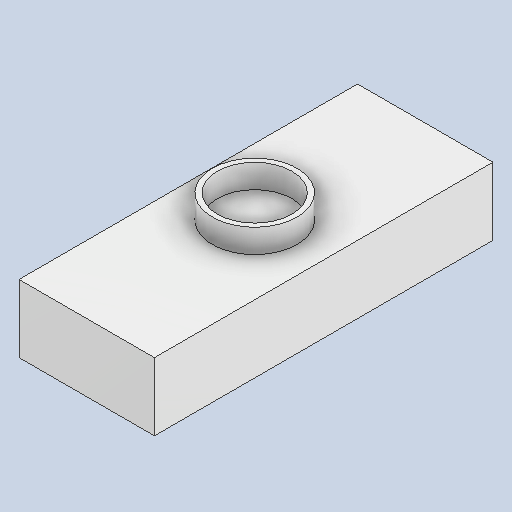
# Autodesk Inventor part: Suporte para estrutura_CPY_CPY1
Saved by Autodesk Inventor 2024 (Build 280153000, 153)
## iProperties
Created: 2024-05-09
Part Number: Suporte para estrutura_CPY_CPY1
Material: ABS plástico
Document SubType Name: Modeling
Designer: mathe
Density: 1.06 g/cm^3
Appearance: Suave - Branco
Author: mathe
Autodesk Inventor part; units mm, degrees
ref_plane "YZ Plane" through (0, 0, 0) normal (1, 0, 0) x (0, 1, 0)
ref_plane "XZ Plane" through (0, 0, 0) normal (0, 1, 0) x (-1, 0, 0)
ref_plane "XY Plane" through (0, 0, 0) normal (0, 0, 1) x (1, 0, 0)
sketch "Esboço1" plane through (0, 0, 0) normal (0, 1, 0) x (-1, 0, 0)
  line L0 (19.6154, -5.2564) -> (-20.3846, -5.2564)
  line L1 (-20.3846, -5.2564) -> (-20.3846, -105.2564)
  line L2 (-20.3846, -105.2564) -> (19.6154, -105.2564)
  line L3 (19.6154, -105.2564) -> (19.6154, -5.2564)
  point P0 (0, 0)
  dimension "d0" = 40
  dimension "d4" = 100
  constraints: 8 end point, 2 parallel, 1 horizontal, 1 perpendicular
  measures "d0" distance between parallel lines of L1 L3
  measures "d4" distance between parallel lines of L2 L0
extrude "Extrusão1" add sketch "Esboço1" along normal blind 20
sketch "Esboço2" plane through (0, 20, 0) normal (0, 1, 0) x (1, 0, 0)
  circle A0 centre (0, 55.2564) radius 12.5
  circle A1 centre (0, 55.2564) radius 11
  line L0 (20.3846, 105.2564) -> (-19.6154, 105.2564) projected
  point P0 (0, 0)
  dimension "d11" = 22
  dimension "d12" = 25
  dimension "d13" = 50
  constraints: 2 centre point, 1 coincident
  measures "d11" diameter of A1
  measures "d12" diameter of A0
  measures "d13" distance from line of L0 A0.centre
extrude "Extrusão2" add sketch "Esboço2" along normal blind 7
sketch "Esboço3" plane through (0, 0, 0) normal (0, -1, 0) x (1, 0, 0)
  circle A0 centre (0.3846, -25.2576) radius 2.5
  circle A1 centre (0, -85.2564) radius 2.5
  line L0 (20.3846, -105.2564) -> (-19.6154, -105.2564) projected
  line L1 (20.3846, -5.2564) -> (20.3846, -105.2564) projected
  point P0 (0, 0)
  dimension "d16" = 5
  dimension "d17" = 5
  dimension "d18" = 60
  dimension "d19" = 20
  dimension "d20" = 20
  constraints: 2 centre point
  measures "d16" diameter of A0
  measures "d17" diameter of A1
  measures "d18" distance of A1.centre A0.centre
  measures "d19" distance from line of L0 A1.centre
  measures "d20" distance from line of L1 A0.centre
extrude "Extrusão3" add sketch "Esboço3" along normal blind 5
